Autodesk Fusion 360 part; units mm, degrees
(part 2 of 2)
sketch "XZ motor engrave" plane through (0, 0, 0) normal (0, -1, 0) x (1, 0, 0)
  circle A0 centre (-275, -15.35) radius 14
  circle A1 centre (-259.5, 0.15) radius 1.5
  circle A2 centre (-259.5, -30.85) radius 1.5
  circle A3 centre (-290.5, 0.15) radius 1.5
  circle A4 centre (-290.5, -30.85) radius 1.5
  circle A5 centre (275, -15.35) radius 14
  circle A6 centre (259.5, 0.15) radius 1.5
  circle A7 centre (259.5, -30.85) radius 1.5
  circle A8 centre (290.5, 0.15) radius 1.5
  circle A9 centre (290.5, -30.85) radius 1.5
  circle A10 centre (-275, 28.5) radius 4
  circle A11 centre (275, 28.5) radius 4
  circle A12 centre (-275, 101.5) radius 10
  circle A13 centre (275, 101.5) radius 10
  circle A14 centre (-133, 100) radius 1.5
  circle A15 centre (-133, 60) radius 1.5
  circle A16 centre (-133, 20) radius 1.5
  circle A17 centre (-133, -20) radius 1.5
  circle A18 centre (-133, -60) radius 1.5
  circle A19 centre (-133, -100) radius 1.5
  circle A20 centre (-133, -140) radius 1.5
  circle A21 centre (-133, -180) radius 1.5
  circle A22 centre (-133, -220) radius 1.5
  circle A23 centre (133, 100) radius 1.5
  circle A24 centre (133, 60) radius 1.5
  circle A25 centre (133, 20) radius 1.5
  circle A26 centre (133, -20) radius 1.5
  circle A27 centre (133, -60) radius 1.5
  circle A28 centre (133, -100) radius 1.5
  circle A29 centre (133, -140) radius 1.5
  circle A30 centre (133, -180) radius 1.5
  circle A31 centre (133, -220) radius 1.5
  circle A32 centre (-149, 260) radius 2.5
  circle A33 centre (-117, 260) radius 2.5
  circle A34 centre (149, 260) radius 2.5
  circle A35 centre (117, 260) radius 2.5
  circle A36 centre (-149, -260) radius 2.5
  circle A37 centre (-117, -260) radius 2.5
  circle A38 centre (149, -260) radius 2.5
  circle A39 centre (117, -260) radius 2.5
  circle A40 centre (242, -225.25) radius 2
  circle A41 centre (242, -125.75) radius 2
  circle A42 centre (242, -26.25) radius 2
  circle A43 centre (-254.5, 52.5) radius 2
  line L0 (-285.5, 56.5) -> (-260.5, 56.5)
  line L1 (-260.5, 56.5) -> (-260.5, 48.5)
  line L2 (-260.5, 48.5) -> (-285.5, 48.5)
  line L3 (-285.5, 48.5) -> (-285.5, 56.5)
  circle A44 centre (-291.5, 52.5) radius 2
  circle A45 centre (254.5, 52.5) radius 2
  line L4 (285.5, 48.5) -> (260.5, 48.5)
  line L5 (260.5, 48.5) -> (260.5, 56.5)
  line L6 (260.5, 56.5) -> (285.5, 56.5)
  line L7 (285.5, 56.5) -> (285.5, 48.5)
  circle A46 centre (291.5, 52.5) radius 2
  circle A47 centre (-254.5, 296) radius 2
  circle A48 centre (-291.5, 296) radius 2
  circle A49 centre (254.5, 296) radius 2
  circle A50 centre (291.5, 296) radius 2
  line L8 (-246, 230) -> (-246, 280)
  line L9 (-246, 280) -> (-238, 280)
  line L10 (-238, 280) -> (-238, 230)
  line L11 (-238, 230) -> (-246, 230)
  line L12 (-246, 149.25) -> (-246, 199.25)
  line L13 (-246, 199.25) -> (-238, 199.25)
  line L14 (-238, 199.25) -> (-238, 149.25)
  line L15 (-238, 149.25) -> (-246, 149.25)
  line L16 (-238, 68.5) -> (-246, 68.5)
  line L17 (-246, 68.5) -> (-246, 118.5)
  line L18 (-246, 118.5) -> (-238, 118.5)
  line L19 (-238, 118.5) -> (-238, 68.5)
  circle A51 centre (-242, 290) radius 2
  circle A52 centre (-242, 58.5) radius 2
  circle A53 centre (-242, 214.625) radius 2
  circle A54 centre (-242, 133.875) radius 2
  line L20 (238, 230) -> (238, 280)
  line L21 (238, 280) -> (246, 280)
  line L22 (246, 280) -> (246, 230)
  line L23 (246, 230) -> (238, 230)
  line L24 (238, 149.25) -> (238, 199.25)
  line L25 (238, 199.25) -> (246, 199.25)
  line L26 (246, 199.25) -> (246, 149.25)
  line L27 (246, 149.25) -> (238, 149.25)
  line L28 (238, 118.5) -> (246, 118.5)
  line L29 (246, 118.5) -> (246, 68.5)
  line L30 (246, 68.5) -> (238, 68.5)
  line L31 (238, 68.5) -> (238, 118.5)
  circle A55 centre (242, 290) radius 2
  circle A56 centre (242, 58.5) radius 2
  circle A57 centre (242, 214.625) radius 2
  circle A58 centre (242, 133.875) radius 2
  line L32 (-246, 48.5) -> (-238, 48.5)
  line L33 (-238, 48.5) -> (-238, -1.5)
  line L34 (-238, -1.5) -> (-246, -1.5)
  line L35 (-246, -1.5) -> (-246, 48.5)
  line L36 (246, -200.5) -> (238, -200.5)
  line L37 (238, -200.5) -> (238, -150.5)
  line L38 (238, -150.5) -> (246, -150.5)
  line L39 (246, -150.5) -> (246, -101)
  line L40 (246, -101) -> (238, -101)
  line L41 (238, -101) -> (238, -51)
  line L42 (238, -51) -> (246, -51)
  line L43 (246, -51) -> (246, -36.5)
  line L44 (246, -36.5) -> (300, -36.5)
  line L45 (300, -36.5) -> (300, 300)
  line L46 (300, 300) -> (285.5, 300)
  line L47 (285.5, 300) -> (285.5, 292)
  line L48 (285.5, 292) -> (260.5, 292)
  line L49 (260.5, 292) -> (260.5, 300)
  line L50 (260.5, 300) -> (-260.5, 300)
  line L51 (-260.5, 300) -> (-260.5, 292)
  line L52 (-260.5, 292) -> (-285.5, 292)
  line L53 (-285.5, 292) -> (-285.5, 300)
  line L54 (-285.5, 300) -> (-300, 300)
  line L55 (-300, 300) -> (-300, -36.5)
  line L56 (-300, -36.5) -> (-246, -36.5)
  line L57 (-246, -36.5) -> (-246, -51)
  line L58 (-246, -51) -> (-238, -51)
  line L59 (-238, -51) -> (-238, -101)
  line L60 (-238, -101) -> (-246, -101)
  line L61 (-246, -101) -> (-246, -150.5)
  line L62 (-246, -150.5) -> (-238, -150.5)
  line L63 (-238, -150.5) -> (-238, -200.5)
  line L64 (-238, -200.5) -> (-246, -200.5)
  line L65 (-246, -200.5) -> (-246, -250)
  line L66 (-246, -250) -> (-238, -250)
  line L67 (-238, -250) -> (-238, -300)
  line L68 (-238, -300) -> (238, -300)
  line L69 (238, -300) -> (238, -250)
  line L70 (238, -250) -> (246, -250)
  line L71 (246, -250) -> (246, -200.5)
  circle A59 centre (-242, -26.25) radius 2
  circle A60 centre (-242, -125.75) radius 2
  circle A61 centre (-242, -225.25) radius 2
  line L72 (238, 48.5) -> (246, 48.5)
  line L73 (246, 48.5) -> (246, -1.5)
  line L74 (246, -1.5) -> (238, -1.5)
  line L75 (238, -1.5) -> (238, 48.5)
  line L76 (253.85, 5.8) -> (300, 5.8)
  line L77 (300, 5.8) -> (300, -36.5)
  line L78 (300, -36.5) -> (253.85, -36.5)
  line L79 (253.85, -36.5) -> (253.85, 5.8)
  circle A62 centre (-133, 140) radius 1.5
  circle A63 centre (133, 140) radius 1.5
  circle A64 centre (-133, 180) radius 1.5
  circle A65 centre (133, 180) radius 1.5
  circle A66 centre (-16, -292.5) radius 2
  circle A67 centre (16, -292.5) radius 2
  circle A68 centre (-133, 220) radius 1.5
  circle A69 centre (133, 220) radius 1.5
  dimension "d160" = 46.15
  dimension "d161" = 42.3
  dimension "d162" = 21.15
  measures "d161" distance of origin
extrude "Extrude14" cut sketch "XZ motor engrave" against normal blind 2 contours L44 L45 L76 L77 L78 L79
mirror "Mirror14" about plane through (0, 0, 0) normal (1, 0, 0) of "Extrude14"
sketch "Y motor holes" plane through (0, 8, 0) normal (0, 1, 0) x (-1, 0, 0)
  circle A0 centre (275, -15.35) radius 14
  circle A1 centre (259.5, 0.15) radius 1.5
  circle A2 centre (259.5, -30.85) radius 1.5
  circle A3 centre (290.5, 0.15) radius 1.5
  circle A4 centre (290.5, -30.85) radius 1.5
  circle A5 centre (-275, -15.35) radius 14
  circle A6 centre (-259.5, 0.15) radius 1.5
  circle A7 centre (-259.5, -30.85) radius 1.5
  circle A8 centre (-290.5, 0.15) radius 1.5
  circle A9 centre (-290.5, -30.85) radius 1.5
  circle A10 centre (275, 28.5) radius 4
  circle A11 centre (-275, 28.5) radius 4
  circle A12 centre (275, 101.5) radius 10
  circle A13 centre (-275, 101.5) radius 10
  circle A14 centre (133, 100) radius 1.5
  circle A15 centre (133, 60) radius 1.5
  circle A16 centre (133, 20) radius 1.5
  circle A17 centre (133, -20) radius 1.5
  circle A18 centre (133, -60) radius 1.5
  circle A19 centre (133, -100) radius 1.5
  circle A20 centre (133, -140) radius 1.5
  circle A21 centre (133, -180) radius 1.5
  circle A22 centre (133, -220) radius 1.5
  circle A23 centre (-133, 100) radius 1.5
  circle A24 centre (-133, 60) radius 1.5
  circle A25 centre (-133, 20) radius 1.5
  circle A26 centre (-133, -20) radius 1.5
  circle A27 centre (-133, -60) radius 1.5
  circle A28 centre (-133, -100) radius 1.5
  circle A29 centre (-133, -140) radius 1.5
  circle A30 centre (-133, -180) radius 1.5
  circle A31 centre (-133, -220) radius 1.5
  circle A32 centre (149, 260) radius 2.5
  circle A33 centre (117, 260) radius 2.5
  circle A34 centre (-149, 260) radius 2.5
  circle A35 centre (-117, 260) radius 2.5
  circle A36 centre (149, -260) radius 2.5
  circle A37 centre (117, -260) radius 2.5
  circle A38 centre (-149, -260) radius 2.5
  circle A39 centre (-117, -260) radius 2.5
  circle A40 centre (-242, -225.25) radius 2
  circle A41 centre (-242, -125.75) radius 2
  circle A42 centre (-242, -26.25) radius 2
  circle A43 centre (242, -225.25) radius 2
  circle A44 centre (242, -125.75) radius 2
  circle A45 centre (242, -26.25) radius 2
  circle A46 centre (-242, 133.875) radius 2
  circle A47 centre (-242, 214.625) radius 2
  circle A48 centre (-242, 58.5) radius 2
  circle A49 centre (-242, 290) radius 2
  line L0 (-246, 118.5) -> (-238, 118.5)
  line L1 (-238, 118.5) -> (-238, 68.5)
  line L2 (-238, 68.5) -> (-246, 68.5)
  line L3 (-246, 68.5) -> (-246, 118.5)
  line L4 (-238, 199.25) -> (-238, 149.25)
  line L5 (-238, 149.25) -> (-246, 149.25)
  line L6 (-246, 149.25) -> (-246, 199.25)
  line L7 (-246, 199.25) -> (-238, 199.25)
  line L8 (-238, 280) -> (-238, 230)
  line L9 (-238, 230) -> (-246, 230)
  line L10 (-246, 230) -> (-246, 280)
  line L11 (-246, 280) -> (-238, 280)
  circle A50 centre (242, 133.875) radius 2
  circle A51 centre (242, 214.625) radius 2
  circle A52 centre (242, 58.5) radius 2
  circle A53 centre (242, 290) radius 2
  line L12 (246, 68.5) -> (238, 68.5)
  line L13 (238, 68.5) -> (238, 118.5)
  line L14 (238, 118.5) -> (246, 118.5)
  line L15 (246, 118.5) -> (246, 68.5)
  line L16 (246, 199.25) -> (246, 149.25)
  line L17 (246, 149.25) -> (238, 149.25)
  line L18 (238, 149.25) -> (238, 199.25)
  line L19 (238, 199.25) -> (246, 199.25)
  line L20 (246, 280) -> (246, 230)
  line L21 (246, 230) -> (238, 230)
  line L22 (238, 230) -> (238, 280)
  line L23 (238, 280) -> (246, 280)
  circle A54 centre (291.5, 296) radius 2
  circle A55 centre (254.5, 296) radius 2
  circle A56 centre (-291.5, 52.5) radius 2
  line L24 (-260.5, 48.5) -> (-285.5, 48.5)
  line L25 (-285.5, 48.5) -> (-285.5, 56.5)
  line L26 (-285.5, 56.5) -> (-260.5, 56.5)
  line L27 (-260.5, 56.5) -> (-260.5, 48.5)
  circle A57 centre (-254.5, 52.5) radius 2
  circle A58 centre (291.5, 52.5) radius 2
  line L28 (260.5, 56.5) -> (285.5, 56.5)
  line L29 (285.5, 56.5) -> (285.5, 48.5)
  line L30 (285.5, 48.5) -> (260.5, 48.5)
  line L31 (260.5, 48.5) -> (260.5, 56.5)
  circle A59 centre (254.5, 52.5) radius 2
  line L32 (-260.5, 300) -> (-260.5, 292)
  line L33 (-260.5, 292) -> (-285.5, 292)
  line L34 (-285.5, 292) -> (-285.5, 300)
  line L35 (-285.5, 300) -> (-300, 300)
  line L36 (-300, 300) -> (-300, -36.5)
  line L37 (-300, -36.5) -> (-246, -36.5)
  line L38 (-246, -36.5) -> (-246, -51)
  line L39 (-238, -300) -> (238, -300)
  line L40 (246, -250) -> (246, -200.5)
  line L41 (246, -36.5) -> (300, -36.5)
  line L42 (300, -36.5) -> (300, 300)
  line L43 (300, 300) -> (285.5, 300)
  line L44 (285.5, 300) -> (285.5, 292)
  line L45 (285.5, 292) -> (260.5, 292)
  line L46 (260.5, 292) -> (260.5, 300)
  line L47 (260.5, 300) -> (-260.5, 300)
  circle A60 centre (-254.5, 296) radius 2
  circle A61 centre (-291.5, 296) radius 2
  line L48 (-15.5, 263.35) -> (15.5, 263.35) construction
  line L49 (15.5, 263.35) -> (15.5, 294.35) construction
  line L50 (15.5, 294.35) -> (-15.5, 294.35) construction
  line L51 (-15.5, 294.35) -> (-15.5, 263.35) construction
  circle A62 centre (0, 278.85) radius 14
  circle A63 centre (15.5, 294.35) radius 1.5
  circle A64 centre (-15.5, 294.35) radius 1.5
  circle A65 centre (-15.5, 263.35) radius 1.5
  circle A66 centre (15.5, 263.35) radius 1.5
  circle A67 centre (133, 140) radius 1.5
  circle A68 centre (-133, 140) radius 1.5
  circle A69 centre (133, 180) radius 1.5
  circle A70 centre (-133, 180) radius 1.5
  circle A71 centre (16, -292.5) radius 2
  circle A72 centre (-16, -292.5) radius 2
  circle A73 centre (133, 220) radius 1.5
  circle A74 centre (-133, 220) radius 1.5
  line L52 (246, -1.5) -> (238, -1.5)
  line L53 (238, -1.5) -> (238, 48.5)
  line L54 (238, 48.5) -> (246, 48.5)
  line L55 (246, 48.5) -> (246, -1.5)
  line L56 (-246, 48.5) -> (-238, 48.5)
  line L57 (-238, 48.5) -> (-238, -1.5)
  line L58 (-238, -1.5) -> (-246, -1.5)
  line L59 (-246, -1.5) -> (-246, 48.5)
  line L60 (-246, -250) -> (-238, -250)
  line L61 (-238, -250) -> (-238, -300)
  line L62 (238, -300) -> (238, -250)
  line L63 (238, -250) -> (246, -250)
  line L64 (246, -200.5) -> (238, -200.5)
  line L65 (238, -200.5) -> (238, -150.5)
  line L66 (238, -150.5) -> (246, -150.5)
  line L67 (246, -150.5) -> (246, -101)
  line L68 (246, -101) -> (238, -101)
  line L69 (238, -101) -> (238, -51)
  line L70 (238, -51) -> (246, -51)
  line L71 (246, -51) -> (246, -36.5)
  line L72 (-246, -51) -> (-238, -51)
  line L73 (-238, -51) -> (-238, -101)
  line L74 (-238, -101) -> (-246, -101)
  line L75 (-246, -101) -> (-246, -150.5)
  line L76 (-246, -150.5) -> (-238, -150.5)
  line L77 (-238, -150.5) -> (-238, -200.5)
  line L78 (-238, -200.5) -> (-246, -200.5)
  line L79 (-246, -200.5) -> (-246, -250)
  dimension "d166" = 31
  dimension "d167" = 31
  dimension "d168" = 28
  dimension "d169" = 3
  dimension "d170" = 3
  dimension "d171" = 3
  dimension "d172" = 3
  dimension "d175" = 21.15
  measures "d168" diameter of A62
  measures "d169" diameter of A63
  measures "d170" diameter of A64
  measures "d171" diameter of A65
  measures "d172" diameter of A66
extrude "Extrude15" cut sketch "Y motor holes" against normal through all contours A62 | A63 | A64 | A65 | A66
sketch "Y motor engrave" plane through (0, 0, 0) normal (0, -1, 0) x (1, 0, 0)
  circle A0 centre (-15.5, 294.35) radius 1.5
  circle A1 centre (0, 278.85) radius 14
  circle A2 centre (-15.5, 263.35) radius 1.5
  circle A3 centre (15.5, 294.35) radius 1.5
  circle A4 centre (15.5, 263.35) radius 1.5
  line L0 (-253.85, 5.8) -> (-253.85, -36.5)
  line L1 (-253.85, -36.5) -> (-246, -36.5)
  line L2 (-246, -36.5) -> (-246, -51)
  line L3 (-246, -51) -> (-238, -51)
  line L4 (-238, -51) -> (-238, -101)
  line L5 (-238, -101) -> (-246, -101)
  line L6 (-246, -101) -> (-246, -150.5)
  line L7 (-246, -150.5) -> (-238, -150.5)
  line L8 (-238, -150.5) -> (-238, -200.5)
  line L9 (-238, -200.5) -> (-246, -200.5)
  line L10 (-246, -200.5) -> (-246, -250)
  line L11 (-246, -250) -> (-238, -250)
  line L12 (-238, -250) -> (-238, -300)
  line L13 (-238, -300) -> (238, -300)
  line L14 (238, -300) -> (238, -250)
  line L15 (238, -250) -> (246, -250)
  line L16 (246, -250) -> (246, -200.5)
  line L17 (246, -200.5) -> (238, -200.5)
  line L18 (238, -200.5) -> (238, -150.5)
  line L19 (238, -150.5) -> (246, -150.5)
  line L20 (246, -150.5) -> (246, -101)
  line L21 (246, -101) -> (238, -101)
  line L22 (238, -101) -> (238, -51)
  line L23 (238, -51) -> (246, -51)
  line L24 (246, -51) -> (246, -36.5)
  line L25 (246, -36.5) -> (253.85, -36.5)
  line L26 (253.85, -36.5) -> (253.85, 5.8)
  line L27 (253.85, 5.8) -> (300, 5.8)
  line L28 (300, 5.8) -> (300, 300)
  line L29 (300, 300) -> (285.5, 300)
  line L30 (285.5, 300) -> (285.5, 292)
  line L31 (285.5, 292) -> (260.5, 292)
  line L32 (260.5, 292) -> (260.5, 300)
  line L33 (260.5, 300) -> (-260.5, 300)
  line L34 (-260.5, 300) -> (-260.5, 292)
  line L35 (-260.5, 292) -> (-285.5, 292)
  line L36 (-285.5, 292) -> (-285.5, 300)
  line L37 (-285.5, 300) -> (-300, 300)
  line L38 (-300, 300) -> (-300, 5.8)
  line L39 (-300, 5.8) -> (-253.85, 5.8)
  line L40 (238, 48.5) -> (246, 48.5)
  line L41 (246, 48.5) -> (246, -1.5)
  line L42 (246, -1.5) -> (238, -1.5)
  line L43 (238, -1.5) -> (238, 48.5)
  circle A5 centre (-242, -225.25) radius 2
  circle A6 centre (-242, -125.75) radius 2
  circle A7 centre (-242, -26.25) radius 2
  line L44 (-246, 48.5) -> (-238, 48.5)
  line L45 (-238, 48.5) -> (-238, -1.5)
  line L46 (-238, -1.5) -> (-246, -1.5)
  line L47 (-246, -1.5) -> (-246, 48.5)
  circle A8 centre (242, 133.875) radius 2
  circle A9 centre (242, 214.625) radius 2
  circle A10 centre (242, 58.5) radius 2
  circle A11 centre (242, 290) radius 2
  line L48 (238, 118.5) -> (246, 118.5)
  line L49 (246, 118.5) -> (246, 68.5)
  line L50 (246, 68.5) -> (238, 68.5)
  line L51 (238, 68.5) -> (238, 118.5)
  line L52 (238, 149.25) -> (238, 199.25)
  line L53 (238, 199.25) -> (246, 199.25)
  line L54 (246, 199.25) -> (246, 149.25)
  line L55 (246, 149.25) -> (238, 149.25)
  line L56 (238, 230) -> (238, 280)
  line L57 (238, 280) -> (246, 280)
  line L58 (246, 280) -> (246, 230)
  line L59 (246, 230) -> (238, 230)
  circle A12 centre (-242, 133.875) radius 2
  circle A13 centre (-242, 214.625) radius 2
  circle A14 centre (-242, 58.5) radius 2
  circle A15 centre (-242, 290) radius 2
  line L60 (-238, 68.5) -> (-246, 68.5)
  line L61 (-246, 68.5) -> (-246, 118.5)
  line L62 (-246, 118.5) -> (-238, 118.5)
  line L63 (-238, 118.5) -> (-238, 68.5)
  line L64 (-246, 149.25) -> (-246, 199.25)
  line L65 (-246, 199.25) -> (-238, 199.25)
  line L66 (-238, 199.25) -> (-238, 149.25)
  line L67 (-238, 149.25) -> (-246, 149.25)
  line L68 (-246, 230) -> (-246, 280)
  line L69 (-246, 280) -> (-238, 280)
  line L70 (-238, 280) -> (-238, 230)
  line L71 (-238, 230) -> (-246, 230)
  circle A16 centre (291.5, 296) radius 2
  circle A17 centre (254.5, 296) radius 2
  circle A18 centre (-291.5, 296) radius 2
  circle A19 centre (-254.5, 296) radius 2
  circle A20 centre (291.5, 52.5) radius 2
  line L72 (285.5, 48.5) -> (260.5, 48.5)
  line L73 (260.5, 48.5) -> (260.5, 56.5)
  line L74 (260.5, 56.5) -> (285.5, 56.5)
  line L75 (285.5, 56.5) -> (285.5, 48.5)
  circle A21 centre (254.5, 52.5) radius 2
  circle A22 centre (-291.5, 52.5) radius 2
  line L76 (-285.5, 56.5) -> (-260.5, 56.5)
  line L77 (-260.5, 56.5) -> (-260.5, 48.5)
  line L78 (-260.5, 48.5) -> (-285.5, 48.5)
  line L79 (-285.5, 48.5) -> (-285.5, 56.5)
  circle A23 centre (-254.5, 52.5) radius 2
  circle A24 centre (242, -26.25) radius 2
  circle A25 centre (242, -125.75) radius 2
  circle A26 centre (242, -225.25) radius 2
  circle A27 centre (117, -260) radius 2.5
  circle A28 centre (149, -260) radius 2.5
  circle A29 centre (-117, -260) radius 2.5
  circle A30 centre (-149, -260) radius 2.5
  circle A31 centre (117, 260) radius 2.5
  circle A32 centre (149, 260) radius 2.5
  circle A33 centre (-117, 260) radius 2.5
  circle A34 centre (-149, 260) radius 2.5
  circle A35 centre (133, -220) radius 1.5
  circle A36 centre (133, -180) radius 1.5
  circle A37 centre (133, -140) radius 1.5
  circle A38 centre (133, -100) radius 1.5
  circle A39 centre (133, -60) radius 1.5
  circle A40 centre (133, -20) radius 1.5
  circle A41 centre (133, 20) radius 1.5
  circle A42 centre (133, 60) radius 1.5
  circle A43 centre (133, 100) radius 1.5
  circle A44 centre (-133, -220) radius 1.5
  circle A45 centre (-133, -180) radius 1.5
  circle A46 centre (-133, -140) radius 1.5
  circle A47 centre (-133, -100) radius 1.5
  circle A48 centre (-133, -60) radius 1.5
  circle A49 centre (-133, -20) radius 1.5
  circle A50 centre (-133, 20) radius 1.5
  circle A51 centre (-133, 60) radius 1.5
  circle A52 centre (-133, 100) radius 1.5
  circle A53 centre (275, 101.5) radius 10
  circle A54 centre (-275, 101.5) radius 10
  circle A55 centre (275, 28.5) radius 4
  circle A56 centre (-275, 28.5) radius 4
  line L80 (21.15, 257.7) -> (-21.15, 257.7)
  line L81 (-21.15, 257.7) -> (-21.15, 300)
  line L82 (-21.15, 300) -> (21.15, 300)
  line L83 (21.15, 300) -> (21.15, 257.7)
  circle A57 centre (133, 140) radius 1.5
  circle A58 centre (-133, 140) radius 1.5
  circle A59 centre (133, 180) radius 1.5
  circle A60 centre (-133, 180) radius 1.5
  circle A61 centre (16, -292.5) radius 2
  circle A62 centre (-16, -292.5) radius 2
  circle A63 centre (133, 220) radius 1.5
  circle A64 centre (-133, 220) radius 1.5
  dimension "d176" = 42.3
  dimension "d177" = 42.3
  dimension "d178" = 21.15
extrude "Extrude16" cut sketch "Y motor engrave" against normal blind 2 contours L33 L80 L81 L82 L83
hole "Hole1" at (-239.4142, 8, 278.5858) direction (0, -1, 0) diameter 4 end up to surface (8 mm away)
hole "Hole2" at (-239.4142, 8, 117.0858) direction (0, -1, 0) diameter 4 end up to surface (8 mm away)
hole "Hole3" at (284.0858, 8, 55.0858) direction (0, -1, 0) diameter 4 end up to surface (8 mm away)
hole "Hole4" at (244.5858, 8, 278.5858) direction (0, -1, 0) diameter 4 end up to surface (8 mm away)
hole "Hole5" at (239.4142, 8, -52.4142) direction (0, -1, 0) diameter 4 end up to surface (8 mm away)
hole "Hole6" at (-239.4142, 8, -0.0858) direction (0, -1, 0) diameter 4 end up to surface (8 mm away)
hole "Hole7" at (239.4142, 8, 150.6642) direction (0, -1, 0) diameter 4 end up to surface (8 mm away)
hole "Hole8" at (244.5858, 8, 197.8358) direction (0, -1, 0) diameter 4 end up to surface (8 mm away)
hole "Hole9" at (-244.5858, 8, 278.5858) direction (0, -1, 0) diameter 4 end up to surface (8 mm away)
hole "Hole10" at (244.5858, 8, 47.0858) direction (0, -1, 0) diameter 4 end up to surface (8 mm away)
hole "Hole11" at (239.4142, 8, 117.0858) direction (0, -1, 0) diameter 4 end up to surface (8 mm away)
hole "Hole12" at (239.4142, 8, -151.9142) direction (0, -1, 0) diameter 4 end up to surface (8 mm away)
hole "Hole13" at (-284.0858, 8, 55.0858) direction (0, -1, 0) diameter 4 end up to surface (8 mm away)
hole "Hole14" at (261.9142, 8, 55.0858) direction (0, -1, 0) diameter 4 end up to surface (8 mm away)
hole "Hole15" at (239.4142, 8, -251.4142) direction (0, -1, 0) diameter 4 end up to surface (8 mm away)
hole "Hole16" at (284.0858, 8, 49.9142) direction (0, -1, 0) diameter 4 end up to surface (8 mm away)
hole "Hole17" at (-244.5858, 8, 47.0858) direction (0, -1, 0) diameter 4 end up to surface (8 mm away)
hole "Hole18" at (244.5858, 8, 69.9142) direction (0, -1, 0) diameter 4 end up to surface (8 mm away)
hole "Hole19" at (-239.4142, 8, 69.9142) direction (0, -1, 0) diameter 4 end up to surface (8 mm away)
hole "Hole20" at (-244.5858, 8, 150.6642) direction (0, -1, 0) diameter 4 end up to surface (8 mm away)
hole "Hole21" at (239.4142, 8, 47.0858) direction (0, -1, 0) diameter 4 end up to surface (8 mm away)
hole "Hole22" at (-239.4142, 8, 231.4142) direction (0, -1, 0) diameter 4 end up to surface (8 mm away)
hole "Hole23" at (-261.9142, 8, 49.9142) direction (0, -1, 0) diameter 4 end up to surface (8 mm away)
hole "Hole24" at (261.9142, 8, 49.9142) direction (0, -1, 0) diameter 4 end up to surface (8 mm away)
hole "Hole25" at (-239.4142, 8, -251.4142) direction (0, -1, 0) diameter 4 end up to surface (8 mm away)
hole "Hole26" at (-244.5858, 8, 69.9142) direction (0, -1, 0) diameter 4 end up to surface (8 mm away)
hole "Hole27" at (-244.5858, 8, -0.0858) direction (0, -1, 0) diameter 4 end up to surface (8 mm away)
hole "Hole28" at (-239.4142, 8, -52.4142) direction (0, -1, 0) diameter 4 end up to surface (8 mm away)
hole "Hole29" at (239.4142, 8, -199.0858) direction (0, -1, 0) diameter 4 end up to surface (8 mm away)
hole "Hole30" at (261.9142, 8, 293.4142) direction (0, -1, 0) diameter 4 end up to surface (8 mm away)
hole "Hole31" at (-244.5858, 8, 117.0858) direction (0, -1, 0) diameter 4 end up to surface (8 mm away)
hole "Hole32" at (239.4142, 8, 197.8358) direction (0, -1, 0) diameter 4 end up to surface (8 mm away)
hole "Hole33" at (-239.4142, 8, 47.0858) direction (0, -1, 0) diameter 4 end up to surface (8 mm away)
hole "Hole34" at (284.0858, 8, 293.4142) direction (0, -1, 0) diameter 4 end up to surface (8 mm away)
hole "Hole35" at (-239.4142, 8, -151.9142) direction (0, -1, 0) diameter 4 end up to surface (8 mm away)
hole "Hole36" at (-239.4142, 8, 197.8358) direction (0, -1, 0) diameter 4 end up to surface (8 mm away)
hole "Hole37" at (239.4142, 8, -99.5858) direction (0, -1, 0) diameter 4 end up to surface (8 mm away)
hole "Hole38" at (-239.4142, 8, -199.0858) direction (0, -1, 0) diameter 4 end up to surface (8 mm away)
hole "Hole39" at (244.5858, 8, -0.0858) direction (0, -1, 0) diameter 4 end up to surface (8 mm away)
hole "Hole40" at (244.5858, 8, 117.0858) direction (0, -1, 0) diameter 4 end up to surface (8 mm away)
hole "Hole41" at (244.5858, 8, 231.4142) direction (0, -1, 0) diameter 4 end up to surface (8 mm away)
hole "Hole42" at (-284.0858, 8, 49.9142) direction (0, -1, 0) diameter 4 end up to surface (8 mm away)
hole "Hole43" at (-261.9142, 8, 55.0858) direction (0, -1, 0) diameter 4 end up to surface (8 mm away)
hole "Hole44" at (-261.9142, 8, 293.4142) direction (0, -1, 0) diameter 4 end up to surface (8 mm away)
hole "Hole45" at (239.4142, 8, -0.0858) direction (0, -1, 0) diameter 4 end up to surface (8 mm away)
hole "Hole46" at (-239.4142, 8, 150.6642) direction (0, -1, 0) diameter 4 end up to surface (8 mm away)
hole "Hole47" at (-239.4142, 8, -99.5858) direction (0, -1, 0) diameter 4 end up to surface (8 mm away)
hole "Hole48" at (239.4142, 8, 231.4142) direction (0, -1, 0) diameter 4 end up to surface (8 mm away)
hole "Hole49" at (-284.0858, 8, 293.4142) direction (0, -1, 0) diameter 4 end up to surface (8 mm away)
hole "Hole50" at (-244.5858, 8, 231.4142) direction (0, -1, 0) diameter 4 end up to surface (8 mm away)
hole "Hole51" at (-244.5858, 8, 197.8358) direction (0, -1, 0) diameter 4 end up to surface (8 mm away)
hole "Hole52" at (244.5858, 8, 150.6642) direction (0, -1, 0) diameter 4 end up to surface (8 mm away)
hole "Hole53" at (239.4142, 8, 69.9142) direction (0, -1, 0) diameter 4 end up to surface (8 mm away)
hole "Hole54" at (239.4142, 8, 278.5858) direction (0, -1, 0) diameter 4 end up to surface (8 mm away)
chamfer "Chamfer1" distance 5 angle 45 2 edges at (-300, 5, -36.5) (300, 5, -36.5)
equation "pannel_thickness = 8.00 mm"
equation "d6 = pannel_thickness"
equation "XZ_joint_thickness = 25 mm"
equation "d30 = pannel_thickness"
equation "d32 = XZ_joint_thickness"
equation "d34 = Tslot_diameter"
equation "d53 = pannel_thickness"
equation "d54 = ( 54 mm - XZ_joint_thickness ) / 2"
equation "d55 = ( 54 mm - XZ_joint_thickness ) / 2"
equation "d56 = XZ_joint_thickness"
equation "d64 = Tslot_diameter"
equation "d71 = pannel_thickness / 2"
equation "d72 = pannel_thickness / 2"
equation "d73 = Tslot_diameter"
equation "d74 = Tslot_diameter"
equation "d75 = pannel_thickness / 2"
equation "d76 = pannel_thickness / 2"
equation "d80 = pannel_thickness"
equation "d81 = Square_joint_thickness"
equation "d86 = Tslot_diameter"
equation "d87 = Tslot_diameter"
equation "d88 = Tslot_diameter"
equation "d89 = Tslot_diameter"
equation "d94 = Square_joint_thickness"
equation "d98 = Square_joint_thickness"
equation "d99 = Square_joint_thickness"
equation "d100 = Square_joint_thickness"
equation "Square_joint_thickness = 50 mm"
equation "d105 = pannel_thickness / 2"
equation "d106 = pannel_thickness / 2"
equation "d107 = pannel_thickness / 2"
equation "d108 = Tslot_diameter"
equation "d109 = Tslot_diameter"
equation "d110 = Tslot_diameter"
equation "d160 = 42.3 mm + 3.85 mm"
equation "d162 = ( 42.3 / 2 ) * 1 mm"
equation "d175 = ( 42.3 / 2 ) * 1 mm"
equation "d178 = ( 42.3 / 2 ) * 1 mm"
equation "d1204 = pannel_thickness + 12 mm"
equation "d1205 = pannel_thickness + 12 mm"
equation "Tslot_diameter = 4 mm"
equation "dbToolDia = 4 mm"
equation "dbOffset = 0 mm" comment "Do NOT change formula"
equation "dbRadius = ( dbToolDia + dbOffset ) / 2" comment "Do NOT change formula"
equation "dbMinPercent = 10"
equation "dbHoleOffset = dbRadius / sqrt(2)" comment "Do NOT change formula"
equation "d1649 = dbRadius * 2"
equation "d1651 = dbHoleOffset"
equation "d1652 = dbHoleOffset"
equation "d1654 = dbRadius * 2"
equation "d1656 = dbHoleOffset"
equation "d1657 = dbHoleOffset"
equation "d1659 = dbRadius * 2"
equation "d1661 = dbHoleOffset"
equation "d1662 = dbHoleOffset"
equation "d1664 = dbRadius * 2"
equation "d1666 = dbHoleOffset"
equation "d1667 = dbHoleOffset"
equation "d1669 = dbRadius * 2"
equation "d1671 = dbHoleOffset"
equation "d1672 = dbHoleOffset"
equation "d1674 = dbRadius * 2"
equation "d1676 = dbHoleOffset"
equation "d1677 = dbHoleOffset"
equation "d1679 = dbRadius * 2"
equation "d1681 = dbHoleOffset"
equation "d1682 = dbHoleOffset"
equation "d1684 = dbRadius * 2"
equation "d1686 = dbHoleOffset"
equation "d1687 = dbHoleOffset"
equation "d1689 = dbRadius * 2"
equation "d1691 = dbHoleOffset"
equation "d1692 = dbHoleOffset"
equation "d1694 = dbRadius * 2"
equation "d1696 = dbHoleOffset"
equation "d1697 = dbHoleOffset"
equation "d1699 = dbRadius * 2"
equation "d1701 = dbHoleOffset"
equation "d1702 = dbHoleOffset"
equation "d1704 = dbRadius * 2"
equation "d1706 = dbHoleOffset"
equation "d1707 = dbHoleOffset"
equation "d1709 = dbRadius * 2"
equation "d1711 = dbHoleOffset"
equation "d1712 = dbHoleOffset"
equation "d1714 = dbRadius * 2"
equation "d1716 = dbHoleOffset"
equation "d1717 = dbHoleOffset"
equation "d1719 = dbRadius * 2"
equation "d1721 = dbHoleOffset"
equation "d1722 = dbHoleOffset"
equation "d1724 = dbRadius * 2"
equation "d1726 = dbHoleOffset"
equation "d1727 = dbHoleOffset"
equation "d1729 = dbRadius * 2"
equation "d1731 = dbHoleOffset"
equation "d1732 = dbHoleOffset"
equation "d1734 = dbRadius * 2"
equation "d1736 = dbHoleOffset"
equation "d1737 = dbHoleOffset"
equation "d1739 = dbRadius * 2"
equation "d1741 = dbHoleOffset"
equation "d1742 = dbHoleOffset"
equation "d1744 = dbRadius * 2"
equation "d1746 = dbHoleOffset"
equation "d1747 = dbHoleOffset"
equation "d1749 = dbRadius * 2"
equation "d1751 = dbHoleOffset"
equation "d1752 = dbHoleOffset"
equation "d1754 = dbRadius * 2"
equation "d1756 = dbHoleOffset"
equation "d1757 = dbHoleOffset"
equation "d1759 = dbRadius * 2"
equation "d1761 = dbHoleOffset"
equation "d1762 = dbHoleOffset"
equation "d1764 = dbRadius * 2"
equation "d1766 = dbHoleOffset"
equation "d1767 = dbHoleOffset"
equation "d1769 = dbRadius * 2"
equation "d1771 = dbHoleOffset"
equation "d1772 = dbHoleOffset"
equation "d1774 = dbRadius * 2"
equation "d1776 = dbHoleOffset"
equation "d1777 = dbHoleOffset"
equation "d1779 = dbRadius * 2"
equation "d1781 = dbHoleOffset"
equation "d1782 = dbHoleOffset"
equation "d1784 = dbRadius * 2"
equation "d1786 = dbHoleOffset"
equation "d1787 = dbHoleOffset"
equation "d1789 = dbRadius * 2"
equation "d1791 = dbHoleOffset"
equation "d1792 = dbHoleOffset"
equation "d1794 = dbRadius * 2"
equation "d1796 = dbHoleOffset"
equation "d1797 = dbHoleOffset"
equation "d1799 = dbRadius * 2"
equation "d1801 = dbHoleOffset"
equation "d1802 = dbHoleOffset"
equation "d1804 = dbRadius * 2"
equation "d1806 = dbHoleOffset"
equation "d1807 = dbHoleOffset"
equation "d1809 = dbRadius * 2"
equation "d1811 = dbHoleOffset"
equation "d1812 = dbHoleOffset"
equation "d1814 = dbRadius * 2"
equation "d1816 = dbHoleOffset"
equation "d1817 = dbHoleOffset"
equation "d1819 = dbRadius * 2"
equation "d1821 = dbHoleOffset"
equation "d1822 = dbHoleOffset"
equation "d1824 = dbRadius * 2"
equation "d1826 = dbHoleOffset"
equation "d1827 = dbHoleOffset"
equation "d1829 = dbRadius * 2"
equation "d1831 = dbHoleOffset"
equation "d1832 = dbHoleOffset"
equation "d1834 = dbRadius * 2"
equation "d1836 = dbHoleOffset"
equation "d1837 = dbHoleOffset"
equation "d1839 = dbRadius * 2"
equation "d1841 = dbHoleOffset"
equation "d1842 = dbHoleOffset"
equation "d1844 = dbRadius * 2"
equation "d1846 = dbHoleOffset"
equation "d1847 = dbHoleOffset"
equation "d1849 = dbRadius * 2"
equation "d1851 = dbHoleOffset"
equation "d1852 = dbHoleOffset"
equation "d1854 = dbRadius * 2"
equation "d1856 = dbHoleOffset"
equation "d1857 = dbHoleOffset"
equation "d1859 = dbRadius * 2"
equation "d1861 = dbHoleOffset"
equation "d1862 = dbHoleOffset"
equation "d1864 = dbRadius * 2"
equation "d1866 = dbHoleOffset"
equation "d1867 = dbHoleOffset"
equation "d1869 = dbRadius * 2"
equation "d1871 = dbHoleOffset"
equation "d1872 = dbHoleOffset"
equation "d1874 = dbRadius * 2"
equation "d1876 = dbHoleOffset"
equation "d1877 = dbHoleOffset"
equation "d1879 = dbRadius * 2"
equation "d1881 = dbHoleOffset"
equation "d1882 = dbHoleOffset"
equation "d1884 = dbRadius * 2"
equation "d1886 = dbHoleOffset"
equation "d1887 = dbHoleOffset"
equation "d1889 = dbRadius * 2"
equation "d1891 = dbHoleOffset"
equation "d1892 = dbHoleOffset"
equation "d1894 = dbRadius * 2"
equation "d1896 = dbHoleOffset"
equation "d1897 = dbHoleOffset"
equation "d1899 = dbRadius * 2"
equation "d1901 = dbHoleOffset"
equation "d1902 = dbHoleOffset"
equation "d1904 = dbRadius * 2"
equation "d1906 = dbHoleOffset"
equation "d1907 = dbHoleOffset"
equation "d1909 = dbRadius * 2"
equation "d1911 = dbHoleOffset"
equation "d1912 = dbHoleOffset"
equation "d1914 = dbRadius * 2"
equation "d1916 = dbHoleOffset"
equation "d1917 = dbHoleOffset"
